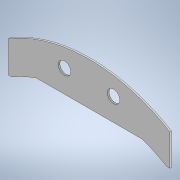
# Autodesk Inventor part: warda
Saved by Autodesk Inventor 2021 (Build 250183000, 183)
## iProperties
Created: 2023-06-18
Part Number: warda
Material: Generic
Document SubType Name: Modeling
Designer: mahmo
Density: 1 g/cm^3
Appearance: Default
Author: mahmo
Autodesk Inventor part; units mm, degrees
ref_plane "YZ Plane" through (0, 0, 0) normal (1, 0, 0) x (0, 1, 0)
ref_plane "XZ Plane" through (0, 0, 0) normal (0, 1, 0) x (-1, 0, 0)
ref_plane "XY Plane" through (0, 0, 0) normal (0, 0, 1) x (1, 0, 0)
sketch "Sketch1" plane through (0, 0, 0) normal (0, 0, 1) x (1, 0, 0)
  circle A0 centre (-7.9561, 43.545) radius 2
  circle A1 centre (7.8751, 43.545) radius 2
  line L0 (-11.8358, 51) -> (11.6369, 51)
  line L1 (-11.8358, 49.5789) -> (-11.8358, 51)
  arc A2 (-11.8358, 49.5789) -> (-25.0147, 44.2928) centre (0, 1) ccw
  line L2 (-25.0147, 44.2928) -> (-26.0147, 44.2928)
  line L3 (-26.0147, 32.5428) -> (-26.0147, 44.2928)
  line L4 (-25.0147, 32.5428) -> (-26.0147, 32.5428)
  arc A3 (-17.1289, 36.2245) -> (-25.0147, 32.5428) centre (0, -10.75) ccw
  line L5 (17.1289, 36.2245) -> (-17.1289, 36.2245)
  arc A4 (25.0147, 32.5428) -> (17.1289, 36.2245) centre (0, -10.75) ccw
  line L6 (25.0147, 32.5428) -> (26.0147, 32.5428)
  line L7 (26.0147, 32.5428) -> (26.0147, 44.2928)
  line L8 (25.0147, 44.2928) -> (26.0147, 44.2928)
  arc A5 (25.0147, 44.2928) -> (11.6369, 49.627) centre (0, 1) ccw
  line L9 (11.6369, 49.627) -> (11.6369, 51)
  circle A6 centre (7.8751, 43.545) radius 2
  circle A7 centre (-7.9561, 43.545) radius 2
  arc A8 (26.0147, 42.6994) -> (-26.0147, 42.6994) centre (0, 0) ccw
  line L10 (-26.0147, 42.6994) -> (-26.0147, 32.5428)
  line L11 (-26.0147, 32.5428) -> (-25.0147, 32.5428)
  arc A9 (-17.1289, 36.2245) -> (-25.0147, 32.5428) centre (0, -10.75) ccw
  line L12 (-17.1289, 36.2245) -> (17.1289, 36.2245)
  arc A10 (25.0147, 32.5428) -> (17.1289, 36.2245) centre (0, -10.75) ccw
  line L13 (26.0147, 32.5428) -> (25.0147, 32.5428)
  line L14 (26.0147, 32.5428) -> (26.0147, 42.6994)
  point P0 (-26.0147, 42.6994)
  point P1 (-25.0147, 32.5428)
  constraints: 30 end point, 14 point on circle, 11 centre point
extrude "Extrusion1" add sketch "Sketch1" along normal blind 0.5 contours A8 L7 L6 A4 L5 A3 L4 L3
body "Solid1"
